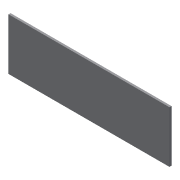
# Autodesk Inventor part: Bottom
Saved by Autodesk Inventor 2016 (Build 200138000, 138)
## iProperties
Created: 2015-05-19
Part Number: Bottom
Material: Generic
Document SubType Name: Modeling
Designer: Andy
Density: 1 g/cm^3
Appearance: Default
Mass: 1948.62 g
Surface Area: 4103.14 cm^2
Volume: 1948.62 cm^3
Author: Andy
Autodesk Inventor part; units mm, degrees
ref_plane "YZ Plane" through (0, 0, 0) normal (1, 0, 0) x (0, 1, 0)
ref_plane "XZ Plane" through (0, 0, 0) normal (0, 1, 0) x (-1, 0, 0)
ref_plane "XY Plane" through (0, 0, 0) normal (0, 0, 1) x (1, 0, 0)
sketch "Sketch1" plane through (0, 0, 0) normal (1, 0, 0) x (0, 1, 0)
  line L0 (0, 0) -> (0, -62)
  line L1 (0, -250) -> (0, 0)
  line L2 (0, 0) -> (0, -62)
  line L3 (10, 0) -> (10, -250)
  line L4 (10, -250) -> (0, -250)
  line L5 (10, 0) -> (0, 0)
  dimension "d4" = 10
  constraints: 12 end point, 1 collinear, 1 horizontal, 1 perpendicular, 1 point on line
  measures "d4" distance between parallel lines of L1 L3
extrude "Extrusion1" add sketch "Sketch1" along normal blind 779.45
body "Solid1"
